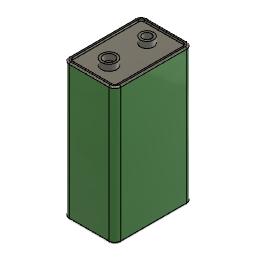
Battery_Mine v1 (Autodesk Fusion 360 design; units mm, degrees)
Autodesk Fusion 360 part; units mm, degrees
sketch "Sketch1" plane through (0, 0, 0) normal (0, 1, 0) x (1, 0, 0)
  line L0 (6.75, 13.25) -> (-6.75, 13.25)
  line L1 (-8.75, 11.25) -> (-8.75, -11.25)
  line L2 (-6.75, -13.25) -> (6.75, -13.25)
  line L3 (8.75, -11.25) -> (8.75, 11.25)
  arc A0 (-6.75, 13.25) -> (-8.75, 11.25) centre (-6.75, 11.25) ccw
  arc A1 (8.75, 11.25) -> (6.75, 13.25) centre (6.75, 11.25) ccw
  arc A2 (6.75, -13.25) -> (8.75, -11.25) centre (6.75, -11.25) ccw
  arc A3 (-8.75, -11.25) -> (-6.75, -13.25) centre (-6.75, -11.25) ccw
  point P0 (8.75, 13.25)
  point P1 (-8.75, 13.25)
  point P2 (8.75, -13.25)
  dimension "d1" = 17.5
  dimension "d2" = 26.5
  dimension "d3" = 2
  constraint horizontal L0
  constraint perpendicular L0 L1
  constraint parallel L0 L2
  constraint parallel L1 L3
  constraint coincident P1 L0
  constraint coincident P1 L1
  constraint tangent L0 A0
  constraint tangent L1 A0
  constraint coincident P0 L0
  constraint coincident P0 L3
  constraint tangent L0 A1
  constraint tangent L3 A1
  constraint equal A0 A1
  constraint coincident P2 L2
  constraint coincident P2 L3
  constraint tangent L2 A2
  constraint tangent L3 A2
  constraint equal A0 A2
  constraint tangent L1 A3
  constraint tangent L2 A3
  constraint equal A0 A3
  measures "d1" distance of P0 P1
  measures "d2" distance of P0 P2
  measures "d3" radius of A0
extrude "Extrude1" add sketch "Sketch1" along normal blind 46.4
sketch "Sketch2" plane through (0, 46.4, 0) normal (0, 1, 0) x (-1, 0, 0)
  arc A0 (8.75, 11.25) -> (6.75, 13.25) centre (6.75, 11.25) ccw
  line L0 (6.75, 13.25) -> (-6.75, 13.25)
  arc A1 (-6.75, 13.25) -> (-8.75, 11.25) centre (-6.75, 11.25) ccw
  line L1 (-8.75, 11.25) -> (-8.75, -11.25)
  arc A2 (-8.75, -11.25) -> (-6.75, -13.25) centre (-6.75, -11.25) ccw
  line L2 (-6.75, -13.25) -> (6.75, -13.25)
  arc A3 (6.75, -13.25) -> (8.75, -11.25) centre (6.75, -11.25) ccw
  line L3 (8.75, -11.25) -> (8.75, 11.25)
  line L4 (7.75, -11.25) -> (7.75, 11.25)
  arc A4 (7.75, 11.25) -> (6.75, 12.25) centre (6.75, 11.25) ccw
  line L5 (6.75, 12.25) -> (-6.75, 12.25)
  arc A5 (-6.75, 12.25) -> (-7.75, 11.25) centre (-6.75, 11.25) ccw
  line L6 (-7.75, 11.25) -> (-7.75, -11.25)
  arc A6 (-7.75, -11.25) -> (-6.75, -12.25) centre (-6.75, -11.25) ccw
  line L7 (-6.75, -12.25) -> (6.75, -12.25)
  arc A7 (6.75, -12.25) -> (7.75, -11.25) centre (6.75, -11.25) ccw
  dimension "d6" = -1
extrude "Extrude2" cut sketch "Sketch2" against normal blind 0.75 contours L4 A4 L5 A5 L6 A6 L7 A7
fillet "Fillet1" radius 0.5 16 edges at (0, 46.4, -13.25) (-8.1642, 46.4, -12.6642) (-8.75, 46.4, 0) (-8.1642, 46.4, 12.6642) (0, 46.4, 13.25) (8.1642, 46.4, 12.6642) (8.75, 46.4, 0) (8.1642, 46.4, -12.6642) (0, 0, -13.25) (-8.1642, 0, -12.6642) (-8.75, 0, 0) (-8.1642, 0, 12.6642) (0, 0, 13.25) (8.1642, 0, 12.6642) (8.75, 0, 0) (8.1642, 0, -12.6642)
sketch "Sketch3" plane through (0, 45.65, 0) normal (0, 1, 0) x (-1, 0, 0)
  arc A0 (6.75, -12.25) -> (7.75, -11.25) centre (6.75, -11.25) ccw
  line L0 (7.75, -11.25) -> (7.75, 11.25)
  arc A1 (7.75, 11.25) -> (6.75, 12.25) centre (6.75, 11.25) ccw
  line L1 (6.75, 12.25) -> (-6.75, 12.25)
  arc A2 (-6.75, 12.25) -> (-7.75, 11.25) centre (-6.75, 11.25) ccw
  line L2 (-7.75, 11.25) -> (-7.75, -11.25)
  arc A3 (-7.75, -11.25) -> (-6.75, -12.25) centre (-6.75, -11.25) ccw
  line L3 (-6.75, -12.25) -> (6.75, -12.25)
  circle A4 centre (0, -6.475) radius 2.25
  circle A5 centre (0, 6.475) radius 2.6
  circle A6 centre (0, -6.475) radius 1.5
  circle A7 centre (0, 6.475) radius 1.9
  dimension "d11" = 6.475
  dimension "d12" = 6.475
  dimension "d13" = 4.5
  dimension "d14" = 5.2
  dimension "d15" = -0.75
  dimension "d16" = -0.7
  measures "d11" distance of origin A4.centre
  measures "d12" distance of origin A5.centre
  measures "d13" diameter of A4
  measures "d14" diameter of A5
extrude "Extrude3" add sketch "Sketch3" along normal blind 2.1 contours A4 | A5
equation "d11 = ( 12.95 / 2 ) * 1 mm"
equation "d12 = ( 12.95 / 2 ) * 1 mm"
